Autodesk Fusion 360 part; units mm, degrees
(part 2 of 2)
equation "d167 = Thickness"
equation "d169 = Thickness"
equation "d171 = Thickness"
equation "d173 = Thickness"
equation "d175 = Tool_diameter"
equation "d176 = Tool_diameter"
equation "d177 = Tool_diameter"
equation "d178 = Tool_diameter"
equation "d184 = Thickness"
equation "d186 = Thickness"
equation "d188 = Thickness"
equation "d190 = Thickness"
equation "d192 = Tool_diameter"
equation "d193 = Tool_diameter"
equation "d194 = Tool_diameter"
equation "d195 = Tool_diameter"
equation "d197 = Thickness"
equation "d199 = Thickness"
equation "d201 = Thickness"
equation "d203 = Thickness"
equation "d205 = Tool_diameter"
equation "d206 = Tool_diameter"
equation "d207 = Tool_diameter"
equation "d208 = Tool_diameter"
equation "d210 = Thickness"
equation "d212 = Thickness"
equation "d214 = Thickness"
equation "d216 = Thickness"
equation "d218 = Tool_diameter"
equation "d219 = Tool_diameter"
equation "d220 = Tool_diameter"
equation "d221 = Tool_diameter"
equation "d223 = Thickness"
equation "d225 = Thickness"
equation "d227 = Thickness"
equation "d229 = Thickness"
equation "d231 = Tool_diameter"
equation "d232 = Tool_diameter"
equation "d233 = Tool_diameter"
equation "d234 = Tool_diameter"
equation "d240 = Thickness"
equation "d242 = Thickness"
equation "d244 = Thickness"
equation "d246 = Thickness"
equation "d248 = Tool_diameter"
equation "d249 = Tool_diameter"
equation "d250 = Tool_diameter"
equation "d251 = Tool_diameter"
equation "d253 = Thickness"
equation "d255 = Thickness"
equation "d257 = Thickness"
equation "d259 = Thickness"
equation "d261 = Tool_diameter"
equation "d262 = Tool_diameter"
equation "d263 = Tool_diameter"
equation "d264 = Tool_diameter"
equation "d266 = Thickness"
equation "d268 = Thickness"
equation "d270 = Thickness"
equation "d272 = Thickness"
equation "d274 = Tool_diameter"
equation "d275 = Tool_diameter"
equation "d276 = Tool_diameter"
equation "d277 = Tool_diameter"
equation "d279 = Thickness"
equation "d281 = Thickness"
equation "d283 = Thickness"
equation "d285 = Thickness"
equation "d287 = Tool_diameter"
equation "d288 = Tool_diameter"
equation "d289 = Tool_diameter"
equation "d290 = Tool_diameter"
equation "d296 = Thickness"
equation "d298 = Thickness"
equation "d300 = Thickness"
equation "d302 = Thickness"
equation "d304 = Tool_diameter"
equation "d305 = Tool_diameter"
equation "d306 = Tool_diameter"
equation "d307 = Tool_diameter"
equation "d309 = Thickness"
equation "d311 = Thickness"
equation "d313 = Thickness"
equation "d315 = Thickness"
equation "d317 = Tool_diameter"
equation "d318 = Tool_diameter"
equation "d319 = Tool_diameter"
equation "d320 = Tool_diameter"
equation "d322 = Thickness"
equation "d324 = Thickness"
equation "d326 = Thickness"
equation "d328 = Thickness"
equation "d330 = Tool_diameter"
equation "d331 = Tool_diameter"
equation "d332 = Tool_diameter"
equation "d333 = Tool_diameter"
equation "d335 = Thickness"
equation "d337 = Thickness"
equation "d339 = Thickness"
equation "d341 = Thickness"
equation "d343 = Tool_diameter"
equation "d344 = Tool_diameter"
equation "d345 = Tool_diameter"
equation "d346 = Tool_diameter"
named bodies: "b  stock body", "b top  body", "b top circles cheese body", "b front  body", "b front circles cheese body", "b back  body", "b back circles cheese body", "b left  body", "b left circles cheese body", "b right  body", "b right circles cheese body", "b bottom  body", "b bottom circles cheese body"
